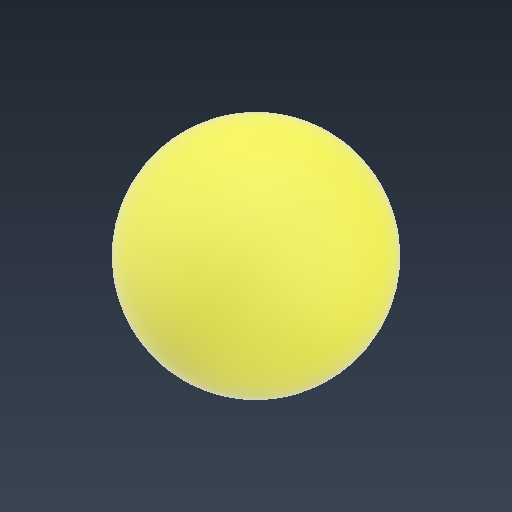
# Autodesk Inventor part: FUEL
Saved by Autodesk Inventor 2026 (Build 300175050, 175E)
## iProperties
Created: 2026-02-08
Part Number: FUEL
Material: Rubber, Butyl
Document SubType Name: Modeling
Designer: Jthib
Mass: 212.541 g
Surface Area: 707.933 cm^2
Volume: 1771.18 cm^3
Density: 0.12 g/cm^3
Appearance: Smooth - Yellow
Author: Jthib
Autodesk Inventor part; units mm, degrees
ref_plane "YZ Plane" through (0, 0, 0) normal (1, 0, 0) x (0, 1, 0)
ref_plane "XZ Plane" through (0, 0, 0) normal (0, 1, 0) x (-1, 0, 0)
ref_plane "XY Plane" through (0, 0, 0) normal (0, 0, 1) x (1, 0, 0)
sketch "Sketch1" plane through (0, 0, 0) normal (0, 0, 1) x (1, 0, 0)
  circle A0 centre (0, 0) radius 75.057
  line L0 (57.7038, 47.9982) -> (-57.7038, -47.9982)
  dimension "d0" = 150.114
  constraints: 2 end point, 2 point on circle, 1 centre point, 1 coincident, 1 midpoint
  measures "d0" diameter of A0
revolve "Revolution1" add sketch "Sketch1" angle 360 about axis through (57.7038, 47.9982, 0) along (-0.7687991, -0.6394904, 0) picked at (-27.2818, 33.6683) contours L0 A0
body "Solid1"
